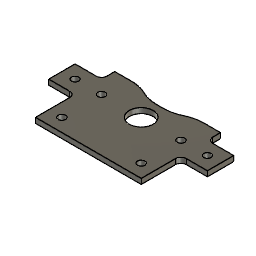
transmitter_support_rxclose (Autodesk Fusion 360 design; units mm, degrees)
Autodesk Fusion 360 part; units mm, degrees
note: some values were not read from the file. Chosen so that the rebuilt part matches the saved one: which bodies a step acts on; which face or edge a step refers to.
sketch "Sketch1" plane through (0, 0, 0) normal (0, 0, 1) x (1, 0, 0)
  line L0 (0, 0) -> (40, 0)
  line L1 (40, 0) -> (40, 40)
  line L2 (40, 40) -> (0, 40)
  line L3 (0, 40) -> (0, 0)
  circle A0 centre (5, 5) radius 1.4
  circle A1 centre (35, 5) radius 1.4
  circle A2 centre (5, 20) radius 1.4
  circle A3 centre (35, 20) radius 1.4
  circle A4 centre (20, 20) radius 4.5
  dimension "d1" = 40
  dimension "d2" = 40
  dimension "d5" = 30
  dimension "d6" = 15
  dimension "d7" = 5
  dimension "d8" = 5
  dimension "d9" = 2.8
  dimension "d10" = 9
  dimension "d11" = 20
  dimension "d12" = 20
  constraint horizontal L0
  constraint vertical L1
  constraint horizontal L2
  constraint vertical L3
  constraint coincident L0.start L3.end
  measures "d1" distance of L0.start L0.end
  measures "d2" distance of L0.end L1.end
  measures "d7" distance of L3 A0.centre
  measures "d8" distance of L0 A0.centre
  measures "d9" diameter of A0
  measures "d10" diameter of A4
  measures "d11" distance of L2 A4.centre
  measures "d12" distance of L1 A4.centre
extrude "Extrude1" add sketch "Sketch1" along normal blind 7 makes body 1
sketch "Sketch2" plane through (0, 0, 7) normal (0, 0, 1) x (-1, 0, 0)
  circle A0 centre (-35, -5) radius 1.4
  circle A1 centre (-20, -20) radius 4.5
  circle A2 centre (-5, -5) radius 1.4
  circle A3 centre (-35, -20) radius 1.4
  circle A4 centre (-5, -20) radius 1.4
  line L0 (0, -40) -> (0, 0)
  line L1 (0, 0) -> (-40, 0)
  line L2 (-40, 0) -> (-40, -40)
  line L3 (-40, -40) -> (0, -40)
  circle A5 centre (-20, -20) radius 4.5
  circle A6 centre (-20, -20) radius 6.25
  dimension "d15" = 12.5
  dimension "d16" = 9
  constraint concentric A1 A5
  constraint concentric A5 A6
  measures "d15" diameter of A6
  measures "d16" diameter of A5
extrude "Extrude2" add sketch "Sketch2" along normal blind 11 contours A6 bodies 1
fillet "Fillet1" radius 2 1 edges at (25.827, 17.7399, 7) on bodies 1
ref_plane "WorkPlane1" through (20, 20, 23) normal (0, 0, 1) x (-1, 0, 0)
sketch "Sketch4" plane through (0, 0, 0) normal (0, 0, -1) x (1, 0, 0)
  circle A0 centre (5, -5) radius 1.4
  circle A1 centre (5, -20) radius 1.4
  circle A2 centre (35, -20) radius 1.4
  circle A3 centre (20, -20) radius 4.5
  circle A4 centre (35, -5) radius 1.4
  line L0 (0, 0) -> (0, -40)
  line L1 (0, -40) -> (40, -40)
  line L2 (40, -40) -> (40, 0)
  line L3 (40, 0) -> (0, 0)
  line L4 (7.5, -3) -> (32.5, -3)
  line L5 (32.5, -3) -> (32.5, -37)
  line L6 (32.5, -37) -> (7.5, -37)
  line L7 (7.5, -37) -> (7.5, -3)
  point P0 (20, -20)
  point P1 (20, -20)
  dimension "d30" = 25
  dimension "d31" = 34
  dimension "d32" = 17
  dimension "d33" = 12.5
  constraint horizontal L4
  constraint vertical L5
  constraint horizontal L6
  constraint vertical L7
  measures "d30" distance of L4.start L4.end
  measures "d31" distance of L4.end L5.end
  measures "d32" distance of L4 P1
  measures "d33" distance of L5 P1
extrude "Extrude4" cut sketch "Sketch4" against normal blind 3 contours L4 L5 L6 L7 bodies 1
fillet "Fillet3" radius 2 4 edges at (20, 37, 3) (32.5, 20, 3) (20, 3, 3) (7.5, 20, 3) on bodies 1
sketch "Sketch5" plane through (0, 0, 18) normal (0, 0, 1) x (-1, 0, 0)
  circle A0 centre (-20, -20) radius 4.5
  circle A1 centre (-20, -20) radius 6.25
  circle A2 centre (-20, -20) radius 4.75
  circle A3 centre (-20, -20) radius 5
  circle A4 centre (-20, -20) radius 5.5
  dimension "d38" = 9.5
  dimension "d41" = 10
  dimension "d44" = 11
  constraint concentric A0 A2
  constraint concentric A2 A3
  constraint concentric A2 A4
  measures "d38" diameter of A2
  measures "d41" diameter of A3
  measures "d44" diameter of A4
extrude "Extrude5" cut sketch "Sketch5" against normal blind 3 contours A2 bodies 1
extrude "Extrude6" cut sketch "Sketch5" against normal blind 2 contours A3 bodies 1
extrude "Extrude7" cut sketch "Sketch5" against normal blind 1 contours A4 bodies 1
sketch "Sketch6" plane through (0, 0, 0) normal (0, 0, 1) x (1, 0, 0)
  line L0 (-60, 35) -> (-20, 35)
  line L1 (-20, 35) -> (-20, 10)
  line L2 (-20, 10) -> (-60, 10)
  line L3 (-60, 10) -> (-60, 35)
  circle A0 centre (-55, 22.5) radius 1.35
  circle A1 centre (-25, 22.5) radius 1.35
  dimension "d47" = 40
  dimension "d48" = 25
  dimension "d49" = 20
  dimension "d50" = 10
  dimension "d78" = 2.7
  dimension "d79" = 5
  dimension "d80" = 12.5
  dimension "d83" = 30
  dimension "d84" = 0
  constraint horizontal L0
  constraint vertical L1
  constraint horizontal L2
  constraint vertical L3
  measures "d47" distance of L1.end L2.end
  measures "d48" distance of L0.end L1.end
  measures "d49" distance of origin L1
  measures "d50" distance of origin L2
  measures "d78" diameter of A0
  measures "d79" distance of L3 A0.centre
  measures "d80" distance of L2 A0.centre
extrude "Extrude8" add sketch "Sketch6" along normal blind 3 separate body contours L0 L1 L2 L3 | A0 | A1 makes body 2
sketch "Sketch7" plane through (0, 0, 3) normal (0, 0, 1) x (-1, 0, 0)
  line L0 (60, -10) -> (20, -10)
  line L1 (20, -10) -> (20, -35)
  line L2 (20, -35) -> (60, -35)
  line L3 (60, -35) -> (60, -10)
  circle A0 centre (40, -22.5) radius 7.35
  circle A1 centre (40, -22.5) radius 6.5
  point P0 (-20, -20)
  point P1 (-20, -20)
  dimension "d53" = 13
  dimension "d54" = 14.7
  dimension "d55" = 12.5
  dimension "d56" = 20
  constraint concentric A0 A1
  constraint coincident P1 P0
  measures "d53" diameter of A1
  measures "d54" diameter of A0
  measures "d55" distance of L2 A0.centre
  measures "d56" distance of L3 A0.centre
extrude "Extrude9" add sketch "Sketch7" along normal blind 20 contours A0 bodies 2
fillet "Fillet4" radius 3.5 1 edges at (-33.1474, 19.8421, 3) on bodies 2
extrude "Extrude10" cut sketch "Sketch7" against normal up to surface (3 mm away) contours A1 bodies 2
sketch "Sketch8" plane through (0, 0, 23) normal (0, 0, 1) x (-1, 0, 0)
  circle A0 centre (40, -22.5) radius 6.5
  circle A1 centre (40, -22.5) radius 7.35
  circle A2 centre (40, -22.5) radius 4.75
  dimension "d75" = 9.5
  constraint concentric A0 A2
  measures "d75" diameter of A2
extrude "Extrude12" add sketch "Sketch8" against normal blind 11 contours A0 bodies 2
extrude "Extrude13" cut sketch "Sketch6" along normal up to surface (3 mm away) contours A0 | A1 bodies 2
move_body "Move2" bodies 2 to x (1, 0, 0) y (0, 1, 0) z (0, 0, 1) at (60, -2.5, 7)
chamfer "Chamfer1" distance 2 angle 45 1 edges at (26.0601, 22.3505, 7) on bodies 2
chamfer "Chamfer2" distance 0.875 angle 45 1 edges at (24.4286, 21.7177, 19) 1 faces at (14.1252, 20.5589, 19) on bodies 2
sketch "Sketch9" plane through (0, 0, 0) normal (0, 0, -1) x (1, 0, 0)
  line L0 (32.5, -3) -> (32.5, -37)
  line L1 (32.5, -37) -> (7.5, -37)
  line L2 (7.5, -37) -> (7.5, -3)
  line L3 (7.5, -3) -> (32.5, -3)
  circle A0 centre (5, -5) radius 1.4
  circle A1 centre (5, -20) radius 1.4
  circle A2 centre (35, -20) radius 1.4
  circle A3 centre (35, -5) radius 1.4
  line L4 (0, 0) -> (0, -40)
  line L5 (0, -40) -> (40, -40)
  line L6 (40, -40) -> (40, 0)
  line L7 (40, 0) -> (0, 0)
  circle A4 centre (5, -20) radius 2.5
  circle A5 centre (5, -5) radius 2.5
  circle A6 centre (35, -5) radius 2.5
  line L8 (41.9596, -43.025) -> (-13.1667, -43.025)
  line L9 (-13.1667, -43.025) -> (-13.1667, 7.931)
  line L10 (-13.1667, 7.931) -> (41.9596, 7.931)
  line L11 (41.9596, 7.931) -> (41.9596, -43.025)
  circle A7 centre (35, -20) radius 2.5
  dimension "d89" = 5
  dimension "d90" = 5
  dimension "d91" = 5
  dimension "d92" = 5
  constraint concentric A1 A4
  constraint concentric A0 A5
  constraint concentric A3 A6
  constraint horizontal L8
  constraint vertical L9
  constraint horizontal L10
  constraint vertical L11
  constraint concentric A2 A7
  measures "d89" diameter of A4
  measures "d90" diameter of A5
  measures "d91" diameter of A6
  measures "d92" diameter of A7
extrude "Extrude14" cut sketch "Sketch9" against normal blind 3 contours L0 L1 L2 L3 | L4 L5 L6 L7 | L8 L9 L10 L11 bodies 1
sketch "Sketch10" plane through (0, 0, 7) normal (0, 0, 1) x (-1, 0, 0)
  line L0 (0, -40) -> (0, 0)
  line L1 (0, 0) -> (-40, 0)
  line L2 (-40, 0) -> (-40, -40)
  line L3 (-40, -40) -> (0, -40)
  circle A0 centre (-35, -5) radius 1.4
  circle A1 centre (-35, -20) radius 1.4
  circle A2 centre (-5, -20) radius 1.4
  circle A3 centre (-5, -5) radius 1.4
  circle A4 centre (-20, -20) radius 8.25
  line L4 (-40, -25) -> (0, -25)
  circle A5 centre (-20, -20) radius 11.25
  dimension "d96" = 25
  dimension "d97" = 22.5
  constraint coincident L2 L4.start
  constraint coincident L0 L4.end
  constraint perpendicular L0 L4
  constraint concentric A4 A5
  measures "d96" distance of L1 L4
  measures "d97" diameter of A5
split "Split2" by plane through (0, 0, 7) normal (0, 0, 1) bodies 1 makes body 3 at (13.7578, 20.3115, 15)
split "Split3" by plane through (0, 0, 3) normal (0, 0, -1) bodies 1 makes body 4 at (7.4969, 5.1246, 2) makes body 5 at (37.4969, 19.8754, 1) makes body 6 at (7.4969, 20.1246, 2) makes body 7 at (37.4969, 4.8754, 1)
extrude "Extrude17" cut 2 faces at (19.7945, 36.0756, 7) (13.0475, 20.6334, 7) along direction (0, 0, -1) blind 2 on bodies 1 bodies 1
sketch "Sketch12" plane through (0, 0, 5) normal (0, 0, 1) x (-1, 0, 0)
  circle A0 centre (-20, -20) radius 4.5
  line L0 (0, -40) -> (0, 0)
  line L1 (0, 0) -> (-40, 0)
  line L2 (-40, 0) -> (-40, -40)
  line L3 (-40, -40) -> (0, -40)
  circle A1 centre (-35, -5) radius 1.4
  circle A2 centre (-35, -20) radius 1.4
  circle A3 centre (-5, -20) radius 1.4
  circle A4 centre (-5, -5) radius 1.4
  line L4 (0, -30) -> (-40, -30)
  line L5 (10, -25) -> (-50, -25)
  line L6 (-50, -25) -> (-50, -15)
  line L7 (-50, -15) -> (10, -15)
  line L8 (10, -15) -> (10, -25)
  circle A5 centre (5, -20) radius 1.35
  circle A6 centre (-45, -20) radius 1.35
  line L9 (-10, -30) -> (-15, -27.1132)
  line L10 (-15, -27.1132) -> (-25, -27.1132)
  line L11 (-25, -27.1132) -> (-30, -30)
  dimension "d113" = 60
  dimension "d114" = 10
  dimension "d115" = 10
  dimension "d116" = 15
  dimension "d117" = 10
  dimension "d118" = 2.7
  dimension "d119" = 5
  dimension "d120" = 5
  dimension "d123" = -50
  dimension "d124" = 0
  dimension "d131" = 10
  dimension "d132" = 150
  dimension "d133" = 150
  dimension "d134" = 10
  dimension "d135" = 10
  constraint coincident L0 L4.start
  constraint coincident L2 L4.end
  constraint perpendicular L2 L4
  constraint horizontal L5
  constraint vertical L6
  constraint horizontal L7
  constraint vertical L8
  constraint coincident L4 L9.start
  constraint parallel L5 L10
  constraint coincident L4 L11.end
  measures "d113" distance of L6.end L7.end
  measures "d114" distance of L5.start L7.end
  measures "d115" distance of L0 L8
  measures "d116" distance of L1 L7
  measures "d117" distance of L3 L4
  measures "d118" diameter of A5
  measures "d119" distance of L5 A5.centre
  measures "d120" distance of L8 A5.centre
  measures "d131" distance of L9.end L10.end
  measures "d132" angle of L4 L9
  measures "d133" angle of L4 L11
  measures "d134" distance of L4.end L11.end
  measures "d135" distance of L4.start L9.start
extrude "Extrude18" cut sketch "Sketch12" against normal blind 2 contours L0 L2 L3 L4 | L4 L9 L10 L11 bodies 1
extrude "Extrude19" add sketch "Sketch12" against normal blind 2 contours L0 L5 L7 L8 | L2 L5 L6 L7 bodies 1
fillet "Fillet7" radius 2 4 edges at (40, 15, 4) (40, 25, 4) (0, 15, 4) (0, 25, 4) on bodies 1
fillet "Fillet8" radius 14 4 edges at (15, 27.1132, 4) (10, 30, 4) (25, 27.1132, 4) (30, 30, 4) on bodies 1
extrude "Extrude15" [suppressed]
fillet "Fillet5" [suppressed]
split "Split1" [suppressed]
sketch "Sketch11" plane through (0, 0, 10) normal (0, 0, 1) x (-1, 0, 0)
  circle A0 centre (-5, -20) radius 1.35
  circle A1 centre (-35, -20) radius 1.35
  line L0 (0, -7.5) -> (-40, -7.5)
  line L1 (-40, -7.5) -> (-40, -25)
  line L2 (0, -25) -> (0, -7.5)
  circle A2 centre (-20, -20) radius 10.85
  line L3 (-40, -17.5) -> (-30, -7.5)
  line L4 (-10, -7.5) -> (0, -17.5)
  line L5 (-40, -25) -> (-32.8087, -25)
  arc A3 (-28.8676, -26.9231) -> (-11.1324, -26.9231) centre (-20, -20) ccw
  line L6 (-7.1913, -25) -> (0, -25)
  arc A4 (-28.8676, -26.9231) -> (-32.8087, -25) centre (-32.8087, -30) ccw
  arc A5 (-7.1913, -25) -> (-11.1324, -26.9231) centre (-7.1913, -30) ccw
  dimension "d102" = 45
  dimension "d103" = 10
  dimension "d104" = 45
  dimension "d105" = 10
  constraint coincident L1 L3.start
  constraint coincident L0 L3.end
  constraint coincident L0 L4.start
  constraint coincident L2 L4.end
  measures "d102" angle of L1 L3
  measures "d103" distance of L0.end L3.end
  measures "d104" angle of L2 L4
  measures "d105" distance of L0.start L4.start
extrude "Extrude16" [suppressed]
fillet "Fillet6" [suppressed]
hidden bodies 2 3 4 5 6 7
